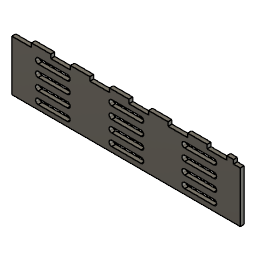
parte trasera intermedio 2-3 piso (Autodesk Fusion 360 design; units mm, degrees)
Autodesk Fusion 360 part; units mm, degrees
sketch "Boceto1" plane through (0, 0, 0) normal (0, 0, 1) x (1, 0, 0)
  line L0 (-117, 26) -> (117, 26)
  line L1 (117, 26) -> (117, -26)
  line L2 (117, -26) -> (-117, -26)
  line L3 (-117, -26) -> (-117, 26)
  line L4 (-117, 26) -> (117, -26) construction
  line L5 (117, 26) -> (-117, -26) construction
  dimension "d1" = 234
  dimension "d2" = 52
  constraint horizontal L0
  constraint perpendicular L0 L1
  constraint parallel L0 L2
  constraint parallel L1 L3
  constraint coincident L4 origin
  constraint coincident L5 origin
  measures "d1" distance of L0.start L0.end
  measures "d2" distance of L0.start L2.end
extrude "Extruir1" add sketch "Boceto1" along normal blind 4
sketch "Boceto2" plane through (0, 0, 4) normal (0, 0, 1) x (1, 0, 0)
  line L0 (-117, -26) -> (117, -26)
  line L1 (117, -26) -> (117, 26)
  line L2 (117, 26) -> (-117, 26)
  line L3 (-117, 26) -> (-117, -26)
  line L4 (-89.9596, 14.7551) -> (-59.9596, 14.7551)
  arc A0 (-59.9596, 14.7551) -> (-59.9596, 20.2449) centre (-59.9596, 17.5) ccw
  line L5 (-59.9596, 20.2449) -> (-89.9596, 20.2449)
  arc A1 (-89.9596, 20.2449) -> (-89.9596, 14.7551) centre (-89.9596, 17.5) ccw
  line L6 (-89.9596, 17.5) -> (-59.9596, 17.5) construction
  arc A2 (-59.9596, 2.7551) -> (-59.9596, 8.2449) centre (-59.9596, 5.5) ccw
  line L7 (-59.9596, 8.2449) -> (-89.9596, 8.2449)
  line L8 (-89.9596, 2.7551) -> (-59.9596, 2.7551)
  arc A3 (-89.9596, 8.2449) -> (-89.9596, 2.7551) centre (-89.9596, 5.5) ccw
  line L9 (-89.9596, 5.5) -> (-59.9596, 5.5) construction
  arc A4 (-59.9596, -9.2449) -> (-59.9596, -3.7551) centre (-59.9596, -6.5) ccw
  line L10 (-59.9596, -3.7551) -> (-89.9596, -3.7551)
  line L11 (-89.9596, -9.2449) -> (-59.9596, -9.2449)
  arc A5 (-89.9596, -3.7551) -> (-89.9596, -9.2449) centre (-89.9596, -6.5) ccw
  line L12 (-89.9596, -6.5) -> (-59.9596, -6.5) construction
  line L13 (-117, 26) -> (117, 26)
  line L14 (-89.9596, -21.2449) -> (-59.9596, -21.2449)
  line L15 (-89.9596, -18.5) -> (-59.9596, -18.5) construction
  line L16 (-59.9596, -15.7551) -> (-89.9596, -15.7551)
  arc A6 (-59.9596, -21.2449) -> (-59.9596, -15.7551) centre (-59.9596, -18.5) ccw
  arc A7 (-89.9596, -15.7551) -> (-89.9596, -21.2449) centre (-89.9596, -18.5) ccw
  line L17 (15.3547, 20.7449) -> (-14.6453, 20.7449)
  arc A8 (15.3547, -20.7449) -> (15.3547, -15.2551) centre (15.3547, -18) ccw
  arc A9 (-14.6453, 8.7449) -> (-14.6453, 3.2551) centre (-14.6453, 6) ccw
  arc A10 (15.3547, -8.7449) -> (15.3547, -3.2551) centre (15.3547, -6) ccw
  line L18 (-14.6453, -6) -> (15.3547, -6) construction
  arc A11 (15.3547, 15.2551) -> (15.3547, 20.7449) centre (15.3547, 18) ccw
  line L19 (-14.6453, 3.2551) -> (15.3547, 3.2551)
  arc A12 (-14.6453, -3.2551) -> (-14.6453, -8.7449) centre (-14.6453, -6) ccw
  line L20 (-14.6453, 18) -> (15.3547, 18) construction
  line L21 (-14.6453, 15.2551) -> (15.3547, 15.2551)
  line L22 (-14.6453, -18) -> (15.3547, -18) construction
  line L23 (15.3547, -3.2551) -> (-14.6453, -3.2551)
  line L24 (-14.6453, 6) -> (15.3547, 6) construction
  arc A13 (-14.6453, -15.2551) -> (-14.6453, -20.7449) centre (-14.6453, -18) ccw
  arc A14 (-14.6453, 20.7449) -> (-14.6453, 15.2551) centre (-14.6453, 18) ccw
  line L25 (-14.6453, -8.7449) -> (15.3547, -8.7449)
  line L26 (15.3547, -15.2551) -> (-14.6453, -15.2551)
  line L27 (-14.6453, -20.7449) -> (15.3547, -20.7449)
  line L28 (15.3547, 8.7449) -> (-14.6453, 8.7449)
  arc A15 (15.3547, 3.2551) -> (15.3547, 8.7449) centre (15.3547, 6) ccw
  line L29 (100, -26) -> (100, 26) construction
  line L30 (117, 26) -> (117, -26)
  arc A16 (59.994, 20.7449) -> (59.994, 15.2551) centre (59.994, 18) ccw
  arc A17 (89.994, 15.2551) -> (89.994, 20.7449) centre (89.994, 18) ccw
  line L31 (59.994, 6) -> (89.994, 6) construction
  line L32 (59.994, 15.2551) -> (89.994, 15.2551)
  line L33 (89.994, 20.7449) -> (59.994, 20.7449)
  arc A18 (59.994, 8.7449) -> (59.994, 3.2551) centre (59.994, 6) ccw
  line L34 (59.994, 3.2551) -> (89.994, 3.2551)
  line L35 (59.994, -6) -> (89.994, -6) construction
  arc A19 (89.994, 3.2551) -> (89.994, 8.7449) centre (89.994, 6) ccw
  line L36 (59.994, -20.7449) -> (89.994, -20.7449)
  line L37 (59.994, -8.7449) -> (89.994, -8.7449)
  arc A20 (59.994, -15.2551) -> (59.994, -20.7449) centre (59.994, -18) ccw
  arc A21 (89.994, -8.7449) -> (89.994, -3.2551) centre (89.994, -6) ccw
  line L38 (59.994, -18) -> (89.994, -18) construction
  arc A22 (89.994, -20.7449) -> (89.994, -15.2551) centre (89.994, -18) ccw
  arc A23 (59.994, -3.2551) -> (59.994, -8.7449) centre (59.994, -6) ccw
  line L39 (89.994, 8.7449) -> (59.994, 8.7449)
  line L40 (89.994, -3.2551) -> (59.994, -3.2551)
  line L41 (59.994, 18) -> (89.994, 18) construction
  line L42 (89.994, -15.2551) -> (59.994, -15.2551)
  point P0 (74.6393, 0)
  dimension "d5" = 30
  dimension "d6" = 30
  dimension "d7" = 30
  dimension "d9" = 8.5
  dimension "d10" = 12
  dimension "d11" = 12
  dimension "d13" = 30
  dimension "d14" = 12
  dimension "d30" = 30
  dimension "d31" = 30
  dimension "d32" = 30
  dimension "d33" = 12
  dimension "d34" = 12
  dimension "d35" = 30
  dimension "d36" = 12
  dimension "d37" = 17
  dimension "d38" = 30
  dimension "d39" = 30
  dimension "d40" = 30
  dimension "d41" = 12
  dimension "d42" = 12
  dimension "d43" = 30
  dimension "d44" = 12
  constraint tangent L4 A0
  constraint tangent A0 L5
  constraint parallel L4 L5
  constraint tangent L5 A1
  constraint tangent L4 A1
  constraint tangent A2 L8
  constraint tangent A2 L7
  constraint parallel L7 L8
  constraint tangent L7 A3
  constraint tangent L8 A3
  constraint tangent A4 L11
  constraint tangent A4 L10
  constraint parallel L10 L11
  constraint tangent L10 A5
  constraint tangent L11 A5
  constraint tangent L14 A6
  constraint tangent L16 A6
  constraint parallel L14 L16
  constraint tangent L16 A7
  constraint tangent L14 A7
  constraint tangent A11 L21
  constraint tangent L17 A11
  constraint parallel L17 L21
  constraint tangent L17 A14
  constraint tangent L21 A14
  constraint tangent L19 A15
  constraint tangent L28 A15
  constraint parallel L19 L28
  constraint tangent A9 L28
  constraint tangent A9 L19
  constraint tangent A10 L25
  constraint tangent A10 L23
  constraint parallel L23 L25
  constraint tangent A12 L23
  constraint tangent A12 L25
  constraint tangent A8 L27
  constraint tangent A8 L26
  constraint parallel L26 L27
  constraint tangent A13 L26
  constraint tangent A13 L27
  constraint coincident L0 L29.start
  constraint coincident L13 L29.end
  constraint tangent A17 L32
  constraint tangent A17 L33
  constraint parallel L32 L33
  constraint tangent A16 L33
  constraint tangent A16 L32
  constraint tangent L34 A19
  constraint tangent A19 L39
  constraint parallel L34 L39
  constraint tangent A18 L39
  constraint tangent A18 L34
  constraint tangent L37 A21
  constraint tangent A21 L40
  constraint parallel L37 L40
  constraint tangent A23 L40
  constraint tangent L37 A23
  constraint tangent L36 A22
  constraint tangent A22 L42
  constraint parallel L36 L42
  constraint tangent A20 L42
  constraint tangent L36 A20
  measures "d5" distance of A1.centre A0.centre
  measures "d6" distance of A2.centre A3.centre
  measures "d7" distance of A4.centre A5.centre
  measures "d9" distance of L6 L13
  measures "d10" distance of L6 L9
  measures "d11" distance of L9 L12
  measures "d13" distance of L15.start L15.end
  measures "d14" distance of L12 L15
  measures "d30" distance of A11.centre L20.start
  measures "d31" distance of A9.centre L24.end
  measures "d32" distance of L18.start A10.centre
  measures "d33" distance of L20 L24
  measures "d34" distance of L18 L24
  measures "d35" distance of A8.centre L22.start
  measures "d36" distance of L18 L22
  measures "d37" distance of L29 L30
  measures "d38" distance of A17.centre A16.centre
  measures "d39" distance of L31.end L31.start
  measures "d40" distance of L35.end L35.start
  measures "d41" distance of L31 L41
  measures "d42" distance of L31 L35
  measures "d43" distance of L38.end A20.centre
  measures "d44" distance of L35 L38
extrude "Extruir2" cut sketch "Boceto2" against normal through all contours L4 A0 L5 A1 | A2 L7 L8 A3 | A4 L10 L11 A5 | L14 L16 A6 A7 | L17 A11 L21 A14 | A8 A13 L26 L27 | A9 L19 L28 A15 | A10 A12 L23 L25 | A16 A17 L32 L33 | A18 L34 A19 L39 | L36 A20 A22 L42 | L37 A21 A23 L40
sketch "Boceto3" plane through (0, 0, 4) normal (0, 0, 1) x (1, 0, 0)
  line L0 (-117, -26) -> (117, -26)
  line L1 (117, -26) -> (117, 26)
  line L2 (117, 26) -> (-117, 26)
  line L3 (-117, 26) -> (-117, -26)
  arc A0 (89.994, -20.7449) -> (89.994, -15.2551) centre (89.994, -18) ccw
  line L4 (89.994, -20.7449) -> (59.994, -20.7449)
  arc A1 (59.994, -15.2551) -> (59.994, -20.7449) centre (59.994, -18) ccw
  line L5 (59.994, -15.2551) -> (89.994, -15.2551)
  arc A2 (-14.6453, -15.2551) -> (-14.6453, -20.7449) centre (-14.6453, -18) ccw
  line L6 (-14.6453, -15.2551) -> (15.3547, -15.2551)
  arc A3 (15.3547, -20.7449) -> (15.3547, -15.2551) centre (15.3547, -18) ccw
  line L7 (15.3547, -20.7449) -> (-14.6453, -20.7449)
  line L8 (-89.9596, -15.7551) -> (-59.9596, -15.7551)
  arc A4 (-59.9596, -21.2449) -> (-59.9596, -15.7551) centre (-59.9596, -18.5) ccw
  line L9 (-59.9596, -21.2449) -> (-89.9596, -21.2449)
  arc A5 (-89.9596, -15.7551) -> (-89.9596, -21.2449) centre (-89.9596, -18.5) ccw
  line L10 (-89.9596, 20.2449) -> (-59.9596, 20.2449)
  arc A6 (-59.9596, 14.7551) -> (-59.9596, 20.2449) centre (-59.9596, 17.5) ccw
  line L11 (-59.9596, 14.7551) -> (-89.9596, 14.7551)
  arc A7 (-89.9596, 20.2449) -> (-89.9596, 14.7551) centre (-89.9596, 17.5) ccw
  line L12 (-14.6453, 20.7449) -> (15.3547, 20.7449)
  arc A8 (15.3547, 15.2551) -> (15.3547, 20.7449) centre (15.3547, 18) ccw
  line L13 (15.3547, 15.2551) -> (-14.6453, 15.2551)
  arc A9 (-14.6453, 20.7449) -> (-14.6453, 15.2551) centre (-14.6453, 18) ccw
  arc A10 (89.994, 15.2551) -> (89.994, 20.7449) centre (89.994, 18) ccw
  line L14 (89.994, 15.2551) -> (59.994, 15.2551)
  arc A11 (59.994, 20.7449) -> (59.994, 15.2551) centre (59.994, 18) ccw
  line L15 (59.994, 20.7449) -> (89.994, 20.7449)
  arc A12 (89.994, -8.7449) -> (89.994, -3.2551) centre (89.994, -6) ccw
  line L16 (89.994, -8.7449) -> (59.994, -8.7449)
  arc A13 (59.994, -3.2551) -> (59.994, -8.7449) centre (59.994, -6) ccw
  line L17 (59.994, -3.2551) -> (89.994, -3.2551)
  arc A14 (-14.6453, -3.2551) -> (-14.6453, -8.7449) centre (-14.6453, -6) ccw
  line L18 (-14.6453, -3.2551) -> (15.3547, -3.2551)
  arc A15 (15.3547, -8.7449) -> (15.3547, -3.2551) centre (15.3547, -6) ccw
  line L19 (15.3547, -8.7449) -> (-14.6453, -8.7449)
  line L20 (-89.9596, -3.7551) -> (-59.9596, -3.7551)
  arc A16 (-59.9596, -9.2449) -> (-59.9596, -3.7551) centre (-59.9596, -6.5) ccw
  line L21 (-59.9596, -9.2449) -> (-89.9596, -9.2449)
  arc A17 (-89.9596, -3.7551) -> (-89.9596, -9.2449) centre (-89.9596, -6.5) ccw
  line L22 (-89.9596, 8.2449) -> (-59.9596, 8.2449)
  arc A18 (-59.9596, 2.7551) -> (-59.9596, 8.2449) centre (-59.9596, 5.5) ccw
  line L23 (-59.9596, 2.7551) -> (-89.9596, 2.7551)
  arc A19 (-89.9596, 8.2449) -> (-89.9596, 2.7551) centre (-89.9596, 5.5) ccw
  line L24 (15.3547, 3.2551) -> (-14.6453, 3.2551)
  arc A20 (-14.6453, 8.7449) -> (-14.6453, 3.2551) centre (-14.6453, 6) ccw
  line L25 (-14.6453, 8.7449) -> (15.3547, 8.7449)
  arc A21 (15.3547, 3.2551) -> (15.3547, 8.7449) centre (15.3547, 6) ccw
  arc A22 (89.994, 3.2551) -> (89.994, 8.7449) centre (89.994, 6) ccw
  line L26 (89.994, 3.2551) -> (59.994, 3.2551)
  arc A23 (59.994, 8.7449) -> (59.994, 3.2551) centre (59.994, 6) ccw
  line L27 (59.994, 8.7449) -> (89.994, 8.7449)
  line L28 (-117, 26) -> (-97, 26)
  line L29 (-97, 30) -> (-77, 30)
  line L30 (-77, 30) -> (-77, 26)
  line L31 (-77, 26) -> (-57, 26)
  line L32 (-57, 30) -> (-37, 30)
  line L33 (-37, 30) -> (-37, 26)
  line L34 (-37, 26) -> (-17, 26)
  line L35 (-17, 30) -> (3, 30)
  line L36 (3, 30) -> (3, 26)
  line L37 (3, 26) -> (23, 26)
  line L38 (23, 30) -> (43, 30)
  line L39 (43, 30) -> (43, 26)
  line L40 (43, 26) -> (63, 26)
  line L41 (63, 30) -> (83, 30)
  line L42 (83, 26) -> (103, 26)
  line L43 (103, 30) -> (103, 26)
  line L44 (-97, 30) -> (-97, 26)
  line L45 (-77, 26) -> (-97, 26)
  line L46 (-57, 30) -> (-57, 26)
  line L47 (-57, 26) -> (-37, 26)
  line L48 (-17, 30) -> (-17, 26)
  line L49 (-17, 26) -> (3, 26)
  line L50 (23, 30) -> (23, 26)
  line L51 (23, 26) -> (43, 26)
  line L52 (63, 30) -> (63, 26)
  line L53 (63, 26) -> (83, 26)
  line L54 (83, 30) -> (83, 26)
  line L55 (103, 30) -> (110, 30)
  line L56 (110, 30) -> (110, 26)
  dimension "d45" = 7
  dimension "d46" = 20
  dimension "d47" = 20
  dimension "d48" = 20
  dimension "d49" = 20
  dimension "d50" = 20
  constraint coincident L2.end L3.start
  constraint coincident L2 L28.end
  constraint perpendicular L3 L29
  constraint coincident L2 L30.end
  constraint perpendicular L2 L30
  constraint coincident L2 L31.end
  constraint perpendicular L30 L32
  constraint coincident L2 L33.end
  constraint perpendicular L2 L33
  constraint coincident L2 L34.end
  constraint perpendicular L33 L35
  constraint coincident L2 L36.end
  constraint perpendicular L2 L36
  constraint coincident L2 L37.end
  constraint perpendicular L36 L38
  constraint coincident L2 L39.end
  constraint perpendicular L2 L39
  constraint coincident L2 L40.end
  constraint perpendicular L39 L41
  constraint coincident L2 L42.start
  constraint coincident L2 L42.end
  constraint perpendicular L42 L43
  constraint perpendicular L28 L44
  constraint perpendicular L2 L46
  constraint perpendicular L34 L48
  constraint perpendicular L37 L50
  constraint perpendicular L40 L52
  constraint parallel L52 L54
  constraint perpendicular L43 L55
  constraint coincident L2 L56.end
  constraint perpendicular L2 L56
  measures "d45" distance of L43.start L55.end
  measures "d46" distance of L41.start L41.end
  measures "d47" distance of L38.start L38.end
  measures "d48" distance of L35.start L35.end
  measures "d49" distance of L32.start L32.end
  measures "d50" distance of L29.start L29.end
extrude "Extruir3" add sketch "Boceto3" against normal blind 4 contours L2 L29 L30 L44 L45 | L2 L43 L55 L56 | L2 L32 L33 L46 L47 | L2 L41 L52 L53 L54 | L2 L35 L36 L48 L49 | L2 L38 L39 L50 L51
